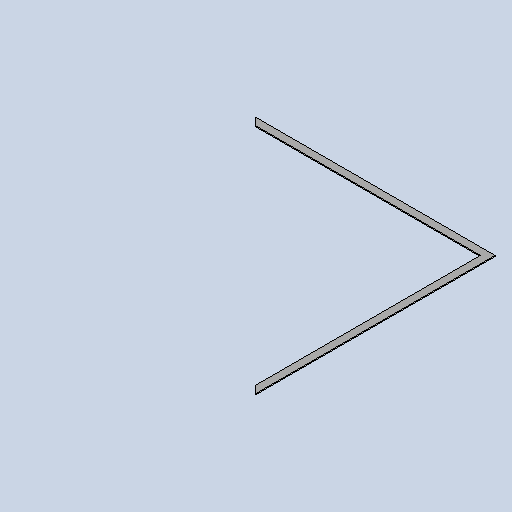
# Autodesk Inventor part: PNS waste water bin 06
Saved by Autodesk Inventor 2025.3 (Build 293356030, 356C)
## iProperties
Created: 2025-09-03
Part Number: PNS waste water bin 06
Material: Generic
Document SubType Name: Sheet Metal
Designer: admin
Density: 1 g/cm^3
Sheet Metal Rule: Default
Appearance: Default
Flat Pattern Width: 48.8293 cm
Flat Pattern Length: 48.8293 cm
Flat Pattern Area: 2384.3 cm^2
Sheet Metal Width: 488,293 mm
Sheet Metal Length: 488,293 mm
Sheet Metal Area: 238429,950 mm^2
Mass: 28.4386 g
Surface Area: 323.105 cm^2
Volume: 28.4386 cm^3
Author: admin
Autodesk Inventor part; units mm, degrees
ref_plane "YZ Plane" through (0, 0, 0) normal (1, 0, 0) x (0, 1, 0)
ref_plane "XZ Plane" through (0, 0, 0) normal (0, 1, 0) x (-1, 0, 0)
ref_plane "XY Plane" through (0, 0, 0) normal (0, 0, 1) x (1, 0, 0)
sketch "Sketch1" plane through (0, 0, 0) normal (0, 0, 1) x (1, 0, 0)
  line L0 (-244.5, 244.5) -> (244.5, 244.5)
  line L1 (244.5, 244.5) -> (244.5, -244.5)
  line L2 (244.5, -244.5) -> (-244.5, -244.5)
  line L3 (-244.5, -244.5) -> (-244.5, 244.5)
  line L4 (-244.5, 244.5) -> (244.5, -244.5) construction
  line L5 (244.5, 244.5) -> (-244.5, -244.5) construction
  line L6 (-229.5, -229.5) -> (229.5, -229.5)
  line L7 (229.5, -229.5) -> (229.5, 229.5)
  line L8 (229.5, 229.5) -> (-229.5, 229.5)
  line L9 (-229.5, 229.5) -> (-229.5, -229.5)
  line L10 (-229.5, -229.5) -> (229.5, 229.5) construction
  line L11 (229.5, -229.5) -> (-229.5, 229.5) construction
  line L12 (-229.5, 229.5) -> (-244.5, 244.5)
  line L13 (229.5, -229.5) -> (244.5, -244.5)
  point P0 (0, 0)
  dimension "d1" = 489
  dimension "d18" = 15
  dimension "d19" = 489
  measures "d1" distance of L0.end L1.end
  measures "d18" distance between parallel lines of L7 L1
  measures "d19" distance of L1.end L2.end
extrude "Plate1" add sketch "Sketch1" along normal blind 2 contours L0 L1 L13 L7 L8 L12
chamfer "Corner Chamfer1" distance 1 angle 45 2 edges at (-244.5, 244.5, 1) (244.5, -244.5, 1)
equation "\"d19\" = d1"
equation "\"d3\" = Thickness"
equation "\"BendRadius\" = Thickness"
equation "\"BendReliefWidth\" = Thickness"
equation "\"BendReliefDepth\" = 0.5 * Thickness"
equation "\"CornerReliefSize\" = 4 * Thickness"
equation "\"MinimumRemnant\" = 2 * Thickness"
equation "\"TransitionRadius\" = BendRadius"
equation "\"JacobiRadiusSize\" = BendRadius"
equation "\"GapSize\" = Thickness"
equation "\"Thickness\" = 2"
body "Solid1"
